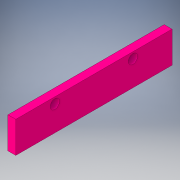
# Autodesk Inventor part: NeoPixel 8 Stick
Saved by Autodesk Inventor 2019 (Build 230136000, 136)
## iProperties
Created: 2019-12-23
Part Number: NeoPixel 8 Stick
Material: Generic
Document SubType Name: Modeling
Designer: james
Density: 1 g/cm^3
Appearance: Default(1)
Author: james
Autodesk Inventor part; units mm, degrees
ref_plane "YZ Plane" through (0, 0, 0) normal (1, 0, 0) x (0, 1, 0)
ref_plane "XZ Plane" through (0, 0, 0) normal (0, 1, 0) x (-1, 0, 0)
ref_plane "XY Plane" through (0, 0, 0) normal (0, 0, 1) x (1, 0, 0)
sketch "Sketch1" plane through (0, 0, 0) normal (1, 0, 0) x (0, 1, 0)
  line L0 (10.2486, 23.6574) -> (0.0886, 23.6574)
  line L1 (0.0886, 23.6574) -> (0.0886, -27.1426)
  line L2 (0.0886, -27.1426) -> (10.2486, -27.1426)
  line L3 (10.2486, -27.1426) -> (10.2486, 23.6574)
  point P0 (0, 0)
  dimension "d0" = 50.8
  dimension "d1" = 10.16
  constraints: 8 end point, 2 parallel, 1 horizontal, 1 perpendicular
  measures "d0" distance of L2.end L0.start
  measures "d1" distance of L0.start L0.end
extrude "Extrusion1" add sketch "Sketch1" along normal blind 2.54
sketch "Sketch2" plane through (2.54, 0, 0) normal (1, 0, 0) x (0, 0, -1)
  line L0 (-23.6574, 0.0886) -> (27.1426, 0.0886) projected
  line L1 (-23.6574, 10.2486) -> (-23.6574, 0.0886) projected
  point P0 (0, 0)
  point P1 (-10.9574, 8.2166)
  point P2 (14.4426, 8.2166)
  dimension "d4" = 0
  dimension "d5" = 8.128
  dimension "d6" = 12.7
  dimension "d7" = 25.4
  measures "d4" vertical distance of point (-10.957, 8.217) point (14.443, 8.217)
  measures "d5" distance from line of L0 point (-10.957, 8.217)
  measures "d6" distance from line of L1 point (-10.957, 8.217)
  measures "d7" distance of point (-10.957, 8.217) point (14.443, 8.217)
hole "Hole1" at (2.54, 8.2166, 10.9574) at (2.54, 8.2166, -14.4426) direction (-1, 0, 0) diameter 3.048 end through all
body "Solid1"
